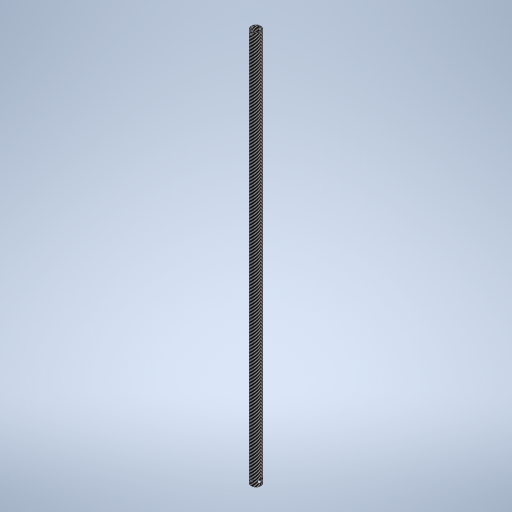
# Autodesk Inventor part: Pendulum Tubing
Saved by Autodesk Inventor 2023 (Build 270158000, 158)
## iProperties
Created: 2023-02-13
Part Number: Pendulum Tubing
Material: Generic
Document SubType Name: Modeling
Designer: mbear
Density: 1 g/cm^3
Appearance: Carbon Fiber
Author: mbear
Autodesk Inventor part; units mm, degrees
ref_plane "XZ Plane" through (0, 0, 0) normal (0, 1, 0) x (-1, 0, 0)
sketch "Sketch1" plane through (0, 0, 0) normal (0, 1, 0) x (-1, 0, 0)
  circle A0 centre (0, 0) radius 6.35
  circle A1 centre (0, 0) radius 5.08
  dimension "d0" = 12.7
  dimension "d1" = 1.27
  constraints: 2 centre point, 2 coincident
  measures "d0" diameter of A0
  measures "d1" radial gap between concentric circles of A1 A0
extrude "Extrusion1" add sketch "Sketch1" along normal blind 508
fillet "Fillet1" radius 0.508 2 edges at (6.35, 508, 0) (5.08, 508, 0)
fillet "Fillet2" radius 0.508 2 edges at (6.35, 0, 0) (5.08, 0, 0)
ref_plane "Work Plane1" through (6.35, 0, 0) normal (1, 0, 0) x (0, 1, 0)
sketch "Sketch2" plane through (6.35, 0, 0) normal (1, 0, 0) x (0, 1, 0)
  circle A0 centre (6.35, 0) radius 3.175
  point P0 (0, 0)
  dimension "d7" = 6.35
  dimension "d8" = 6.35
  constraints: 1 centre point
  measures "d7" diameter of A0
  measures "d8" distance of A0.centre point (0, 0)
extrude "Extrusion2" cut sketch "Sketch2" against normal blind 25.4
ref_plane "Work Plane2" through (0, 0, 6.35) normal (0, 0, 1) x (1, 0, 0)
sketch "Sketch3" plane through (0, 0, 6.35) normal (0, 0, 1) x (1, 0, 0)
  circle A0 centre (0, 6.35) radius 0.6302
  point P0 (0, 0)
  dimension "d12" = 6.35
  constraints: 1 centre point
  measures "d12" distance of point (0, 0) A0.centre
hole "Hole1" at (0, 6.35, 6.35) direction (0, 0, -1) diameter 3.4 depth 25.4 tip angle 118 clearance for "Socket Head Cap Screw" size "M3" standard "Ansi Metric M Profile"
sketch "Sketch5" plane through (0, 0, 6.35) normal (0, 0, 1) x (1, 0, 0)
  circle A0 centre (0, 504.825) radius 3.0853
  line L0 (-5.842, 508) -> (5.842, 508) projected
  point P0 (0, 0)
  dimension "d20" = 3.175
  constraints: 1 centre point
  measures "d20" distance from line of L0 A0.centre
hole "Hole2" at (0, 504.825, 6.35) direction (0, 0, -1) diameter 3.4 depth 25.4 tip angle 118 clearance for "Socket Head Cap Screw" size "M3" standard "Ansi Metric M Profile"
body "Solid1"
